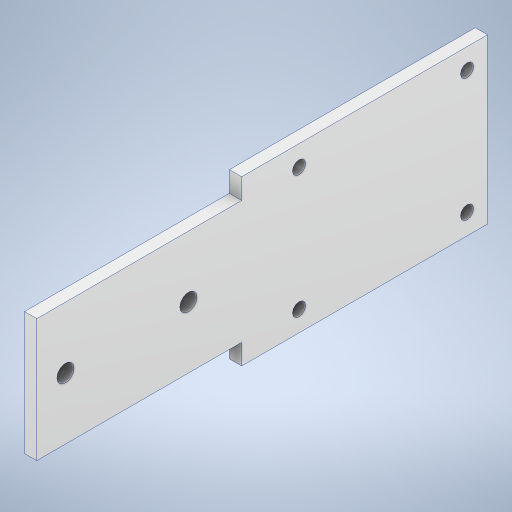
# Autodesk Inventor part: link4_plate1
Saved by Autodesk Inventor 2024 (Build 280153000, 153)
## iProperties
Created: 2024-12-13
Part Number: link4_plate1
Material: アルミニウム 6061
Document SubType Name: Modeling
Designer: hirek
Density: 2.7 g/cm^3
Appearance: アルミニウム - フラット
Mass: 37.9594 g
Surface Area: 106.915 cm^2
Volume: 14.059 cm^3
Author: hirek
Autodesk Inventor part; units mm, degrees
ref_plane "YZ Plane" through (0, 0, 0) normal (1, 0, 0) x (0, 1, 0)
ref_plane "XZ Plane" through (0, 0, 0) normal (0, 1, 0) x (-1, 0, 0)
ref_plane "XY Plane" through (0, 0, 0) normal (0, 0, 1) x (1, 0, 0)
sketch "スケッチ1" plane through (0, 0, 0) normal (1, 0, 0) x (0, 1, 0)
  line L0 (35, -42.2311) -> (-5, -42.2311)
  line L1 (-5, -42.2311) -> (-5, -102.2311)
  line L2 (-5, -102.2311) -> (35, -102.2311)
  line L3 (35, -102.2311) -> (35, -42.2311)
  line L4 (30, 7.7689) -> (0, 7.7689)
  line L5 (0, 7.7689) -> (0, -42.2311)
  line L6 (0, -42.2311) -> (30, -42.2311)
  line L7 (30, -42.2311) -> (30, 7.7689)
  dimension "d1" = 40
  dimension "d2" = 60
  dimension "d68" = 30
  dimension "d69" = 50
  dimension "d70" = 0
  dimension "d71" = 5
  constraints: 16 end point, 4 parallel, 2 horizontal, 2 perpendicular
  measures "d1" distance of L2.end L1.end
  measures "d2" distance of L1.end L0.end
  measures "d68" distance of L6.end L5.end
  measures "d69" distance of L5.end L4.end
  measures "d70" distance between parallel lines of L6 L0
  measures "d71" distance between parallel lines of L7 L3
extrude "押し出し1" add sketch "スケッチ1" along normal blind 3
sketch "スケッチ4" plane through (3, 0, 0) normal (1, 0, 0) x (0, 0, -1)
  line L0 (56.2311, 30) -> (97.2311, 30)
  line L1 (97.2311, 30) -> (97.2311, 0)
  line L2 (97.2311, 0) -> (56.2311, 0)
  line L3 (56.2311, 0) -> (56.2311, 30)
  line L4 (102.2311, 35) -> (42.2311, 35) projected
  line L5 (102.2311, -5) -> (102.2311, 35) projected
  point P0 (0, 0)
  dimension "d29" = 41
  dimension "d30" = 30
  dimension "d31" = 5
  dimension "d32" = 5
  constraints: 8 end point, 4 coincident, 2 parallel, 1 horizontal, 1 perpendicular
  measures "d29" distance of L1.end L2.end
  measures "d30" distance of L0.end L1.end
  measures "d31" distance between parallel lines of L0 L4
  measures "d32" distance between parallel lines of L5 L1
hole "穴2" at (3, 30, -56.2311) at (3, 0, -56.2311) at (3, 0, -97.2311) at (3, 30, -97.2311) direction (-1, 0, 0) diameter 3.2 end through all
sketch "スケッチ7" plane through (3, 0, 0) normal (1, 0, 0) x (0, 0, -1)
  line L0 (102.2311, -5) -> (102.2311, 35) projected
  line L1 (102.2311, 15) -> (-7.7689, 15)
  line L2 (-7.7689, 30) -> (-7.7689, 0) projected
  point P0 (0, 0)
  point P1 (-0.7689, 15)
  point P2 (29.2311, 15)
  dimension "d72" = 7
  dimension "d73" = 30
  constraints: 2 end point, 2 midpoint, 2 point on line
  measures "d72" distance from line of point (-0.769, 15) L2
  measures "d73" distance of point (29.231, 15) point (-0.769, 15)
hole "穴5" at (3, 15, 0.7689) at (3, 15, -29.2311) direction (-1, 0, 0) diameter 4.2 end through all
